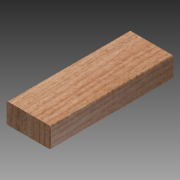
# Autodesk Inventor part: Left Mounting Board 2x4
Saved by Autodesk Inventor 2014 (Build 180170000, 170)
## iProperties
Created: 2016-02-05
Part Number: Left Mounting Board 2x4
Material: Generic
Document SubType Name: Modeling
Designer: zoldberg
Density: 1 g/cm^3
Appearance: Birch - Natural Polished
Author: zoldberg
Autodesk Inventor part; units mm, degrees
ref_plane "YZ Plane" through (0, 0, 0) normal (1, 0, 0) x (0, 1, 0)
ref_plane "XZ Plane" through (0, 0, 0) normal (0, 1, 0) x (-1, 0, 0)
ref_plane "XY Plane" through (0, 0, 0) normal (0, 0, 1) x (1, 0, 0)
sketch "Sketch1" plane through (0, 0, 0) normal (0, 0, 1) x (1, 0, 0)
  line L0 (-41.275, -19.05) -> (41.275, -19.05)
  line L1 (41.275, -19.05) -> (41.275, 19.05)
  line L2 (41.275, 19.05) -> (-41.275, 19.05)
  line L3 (-41.275, 19.05) -> (-41.275, -19.05)
  line L4 (-41.275, -19.05) -> (41.275, 19.05) construction
  line L5 (41.275, -19.05) -> (-41.275, 19.05) construction
  point P0 (0, 0)
  dimension "d0" = 82.55
  dimension "d1" = 38.1
  constraints: 12 end point, 2 midpoint, 2 parallel, 1 horizontal, 1 perpendicular
  measures "d0" distance of L2.end L1.end
  measures "d1" distance of L1.end L0.end
extrude "Extrusion1" add sketch "Sketch1" along normal blind 228.6
fillet "Fillet1" radius 3.175 4 edges at (41.275, 19.05, 114.3) (-41.275, 19.05, 114.3) (41.275, -19.05, 114.3) (-41.275, -19.05, 114.3)
body "Solid1"
